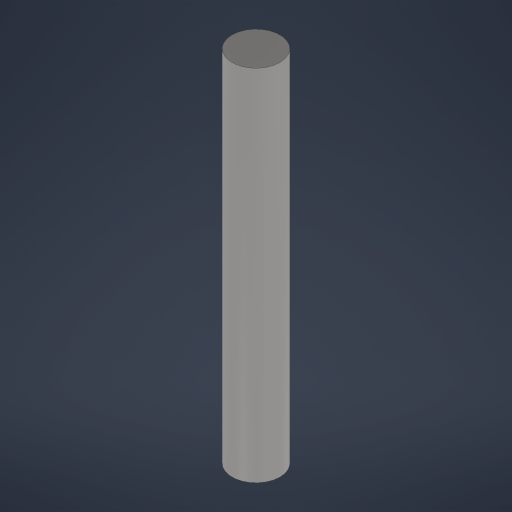
# Autodesk Inventor part: Base-Shaft
Saved by Autodesk Inventor 2023 (Build 270158000, 158)
## iProperties
Created: 2023-09-17
Part Number: Base-Shaft
Material: Steel, Mild
Document SubType Name: Modeling
Designer: Abhinav
Density: 7.85 g/cm^3
Appearance: Semi-Polished
Author: Abhinav
Autodesk Inventor part; units mm, degrees
ref_plane "YZ Plane" through (0, 0, 0) normal (1, 0, 0) x (0, 1, 0)
ref_plane "XZ Plane" through (0, 0, 0) normal (0, 1, 0) x (-1, 0, 0)
ref_plane "XY Plane" through (0, 0, 0) normal (0, 0, 1) x (1, 0, 0)
sketch "Sketch1" plane through (0, 0, 0) normal (0, 1, 0) x (-1, 0, 0)
  circle A0 centre (0, 0) radius 10
  dimension "d0" = 20
  constraints: 1 centre point, 1 coincident
  measures "d0" diameter of A0
extrude "Extrusion1" add sketch "Sketch1" along normal blind 150
body "Solid1"
